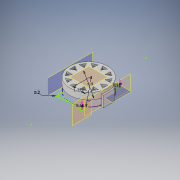
# Autodesk Inventor part: watchBodyOneTopV1.1
Saved by Autodesk Inventor 2019 (Build 230136000, 136)
## iProperties
Created: 2019-10-08
Part Number: watchBodyOneTopV1.1
Material: Generic
Document SubType Name: Modeling
Designer: Derek
Density: 1 g/cm^3
Appearance: Default
Author: Derek
Autodesk Inventor part; units mm, degrees
ref_plane "YZ Plane" through (0, 0, 0) normal (1, 0, 0) x (0, 1, 0)
ref_plane "XZ Plane" through (0, 0, 0) normal (0, 1, 0) x (-1, 0, 0)
ref_plane "XY Plane" through (0, 0, 0) normal (0, 0, 1) x (1, 0, 0)
sketch "Sketch1" plane through (0, 0, 0) normal (0, 1, 0) x (-1, 0, 0)
  circle A0 centre (0, 0) radius 22
  arc A1 (-13.7238, -17.1947) -> (13.7238, -17.1947) centre (0, 0) ccw
  dimension "d0" = 44
  dimension "d11" = 13.7238
  constraints: 4 point on circle, 2 centre point, 1 coincident, 1 concentric
  measures "d0" diameter of A0
  measures "d11" horizontal distance of point (0, 0) A0.start
ref_plane "Work Plane10" through (0, 7, 0) normal (0, 1, 0) x (1, 0, 0)
sketch "Sketch5" plane through (0, 7, 0) normal (0, 1, 0) x (1, 0, 0)
  circle A0 centre (0, 0) radius 20
  dimension "d8" = 40
  constraints: 1 centre point, 1 coincident
  measures "d8" diameter of A0
ref_plane "Work Plane9" through (0, 0, 0) normal (0, -1, 0) x (1, 0, 0)
sketch "Sketch8" plane through (0, 0, 0) normal (0, -1, 0) x (1, 0, 0)
  arc A0 (-11.5874, -18.7011) -> (11.5874, -18.7011) centre (0, 0) ccw
  line L0 (-15.0453, -16.0511) -> (-15.0453, -22.0257)
  line L1 (15.0453, -16.0511) -> (15.0453, -22.0257)
  arc A1 (-15.0453, -16.0511) -> (15.0453, -16.0511) centre (0, 0) ccw
  arc A2 (-15.0453, -22.0257) -> (-13.0453, -24.0257) centre (-13.0453, -22.0257) ccw
  arc A3 (13.0453, -24.0257) -> (15.0453, -22.0257) centre (13.0453, -22.0257) ccw
  line L2 (-15.0451, -16.0514) -> (-15.0451, -22.026)
  arc A4 (-15.0451, -22.026) -> (-13.0451, -24.026) centre (-13.0451, -22.026) ccw
  arc A5 (13.0456, -24.026) -> (15.0456, -22.026) centre (13.0456, -22.026) ccw
  line L3 (15.0456, -16.0514) -> (15.0456, -22.026)
  arc A6 (-15.0451, -16.0514) -> (15.0456, -16.0514) centre (0.0003, -0.0002) ccw
  arc A7 (13.0456, -24.026) -> (-13.0451, -24.026) centre (0.0003, -66.8475) ccw
  point P0 (0, 0)
  point P1 (0, 0)
  constraints: 16 point on circle, 8 centre point, 8 end point
ref_plane "Work Plane8" through (0, 0, 0) normal (0, -1, 0) x (1, 0, 0)
sketch "Sketch11" plane through (0, 0, 0) normal (0, -1, 0) x (1, 0, 0)
  arc A0 (11.5874, 18.7011) -> (-11.5874, 18.7011) centre (0, 0) ccw
  line L0 (-15.0453, 16.0511) -> (-15.0453, 22.0257)
  line L1 (15.0453, 16.0511) -> (15.0453, 22.0257)
  arc A1 (15.0453, 16.0511) -> (-15.0453, 16.0511) centre (0, 0) ccw
  arc A2 (-13.0453, 24.0257) -> (-15.0453, 22.0257) centre (-13.0453, 22.0257) ccw
  arc A3 (15.0453, 22.0257) -> (13.0453, 24.0257) centre (13.0453, 22.0257) ccw
  line L2 (-15.0451, 16.0514) -> (-15.0451, 22.026)
  arc A4 (-13.0451, 24.026) -> (-15.0451, 22.026) centre (-13.0451, 22.026) ccw
  arc A5 (15.0456, 22.026) -> (13.0456, 24.026) centre (13.0456, 22.026) ccw
  line L3 (15.0456, 16.0514) -> (15.0456, 22.026)
  arc A6 (15.0456, 16.0514) -> (-15.0451, 16.0514) centre (0.0003, 0.0002) ccw
  arc A7 (-13.0451, 24.026) -> (13.0456, 24.026) centre (0.0003, 66.8475) ccw
  point P0 (0, 0)
  dimension "d27" = 2
  dimension "d28" = 2
  constraints: 16 point on circle, 8 centre point, 8 end point, 4 tangent, 4 vertical, 2 equal radius
  measures "d27" radius of A2
  measures "d28" radius of A4
ref_plane "Work Plane5" through (14.0456, 0, 22.026) normal (1, 0, 0) x (0, 0, -1)
sketch "Sketch14" plane through (14.0456, 0, 22.026) normal (1, 0, 0) x (0, 0, -1)
  line L0 (0, 0) -> (0, 7) projected
  circle A0 centre (0, 3.5) radius 0.9
  point P0 (22.026, 0)
  dimension "d38" = 1.8
  constraints: 1 centre point, 1 midpoint
  measures "d38" diameter of A0
ref_plane "Work Plane6" through (14.0456, 0, 22.026) normal (1, 0, 0) x (0, 0, -1)
sketch "Sketch15" plane through (14.0456, 0, 22.026) normal (1, 0, 0) x (0, 0, -1)
  line L0 (44.1089, 7) -> (44.1089, 0) projected
  circle A0 centre (44.1089, 3.5) radius 0.9
  point P0 (22.026, 0)
  dimension "d41" = 1.8
  constraints: 1 centre point, 1 midpoint
  measures "d41" diameter of A0
ref_plane "Work Plane7" through (0, 7, 0) normal (0, 1, 0) x (1, 0, 0)
sketch "Sketch16" plane through (0, 7, 0) normal (0, 1, 0) x (1, 0, 0)
  circle A0 centre (0, 0) radius 22
  circle A1 centre (0, -0.3745) radius 18.6
  dimension "d44" = 37.2
  constraints: 2 centre point, 1 coincident
  measures "d44" diameter of A1
extrude "Extrusion13" add sketch "Sketch16" along normal blind 7.5
ref_plane "Work Plane3" through (22, 0, 0) normal (1, 0, 0) x (0, 1, 0)
sketch "Sketch17" plane through (22, 0, 0) normal (1, 0, 0) x (0, 1, 0)
  line L0 (7, -18.2255) -> (7, 18.9745) projected
  line L1 (11.1125, 6.35) -> (7, 6.35)
  line L2 (7, 6.35) -> (7, -6.5465)
  line L3 (7, -6.5465) -> (11.1125, -6.5465)
  line L4 (11.1125, -6.5465) -> (11.1125, 6.35)
  constraints: 8 end point, 2 parallel, 1 horizontal, 1 perpendicular, 1 point on line
extrude "Extrusion14" add sketch "Sketch17" along normal mid plane 3
ref_plane "Work Plane12" through (21.0034, 7, -6.5465) normal (0, -1, 0) x (1, 0, 0)
sketch "Sketch18" plane through (21.0034, 7, -6.5465) normal (0, -1, 0) x (1, 0, 0)
  arc A0 (-35.8073, -9.7276) -> (-35.8073, 22.8206) centre (-21.0034, 6.5465) ccw projected
  line L0 (0, 0) -> (2.4966, 0) projected
  line L1 (0, 0) -> (2.4966, 0)
  line L2 (2.4966, 12.8965) -> (0.0602, 12.8965) projected
  line L3 (2.4966, 0) -> (2.4966, 12.8965)
  line L4 (2.4966, 12.8965) -> (0.0602, 12.8965)
  arc A1 (0, 0) -> (0.0602, 12.8965) centre (-21.0034, 6.5465) ccw
  constraints: 6 end point, 3 point on circle, 2 collinear, 1 centre point, 1 perpendicular
extrude "Extrusion15" add sketch "Sketch18" along normal blind 8.65
ref_plane "Work Plane4" through (-22, 0, 0) normal (-1, 0, 0) x (0, -1, 0)
sketch "Sketch19" plane through (-22, 0, 0) normal (-1, 0, 0) x (0, -1, 0)
  line L0 (-11.1125, -6.5465) -> (-11.1125, 6.35) projected
  line L1 (-7, -20) -> (-7, 20) projected
  line L2 (-11.1125, -6.5465) -> (-7, -6.5465)
  line L3 (-7, -6.5465) -> (-7, 6.35)
  line L4 (-7, 6.35) -> (-11.1125, 6.35)
  line L5 (-11.1125, 6.35) -> (-11.1125, -6.5465)
  point P0 (0, 0)
  constraints: 8 end point, 2 parallel, 1 horizontal, 1 perpendicular, 1 point on line
extrude "Extrusion16" add sketch "Sketch19" along normal mid plane 3
sketch "Sketch20" plane through (-23.5, 7, -6.5465) normal (0, -1, 0) x (1, 0, 0)
  line L0 (0, 0) -> (2.4966, 0) projected
  line L1 (2.4966, 0) -> (0, 0)
  line L2 (0, 12.8965) -> (0, 0) projected
  line L3 (0, 0) -> (0, 12.8965)
  arc A0 (2.4363, 12.8965) -> (2.4966, 0) centre (23.5, 6.5465) ccw projected
  line L4 (0, 12.8965) -> (2.4363, 12.8965)
  point P0 (3, 0)
  constraints: 6 end point, 2 collinear, 1 perpendicular
extrude "Extrusion17" add sketch "Sketch20" along normal blind 8.65
sketch "Sketch21" plane through (-23.5, 0, 0) normal (-1, 0, 0) x (0, 0, 1)
  line L0 (-6.5465, 11.1125) -> (-6.5465, -1.65) projected
  line L1 (6.35, -1.65) -> (-6.5465, -1.65)
  line L2 (-6.5465, -1.65) -> (-6.5465, -0.292)
  line L3 (-6.5465, -0.292) -> (6.35, -0.292)
  line L4 (6.35, -0.292) -> (6.35, -1.65)
  point P0 (6.35, 0)
  constraints: 8 end point, 2 parallel, 1 horizontal, 1 perpendicular, 1 point on line
extrude "Extrusion18" add sketch "Sketch21" against normal blind 3.5
sketch "Sketch22" plane through (23.5, 0, 0) normal (1, 0, 0) x (0, 0, -1)
  line L0 (-6.35, -0.292) -> (6.5465, -0.292) projected
  line L1 (-6.35, -1.65) -> (6.5465, -1.65) projected
  line L2 (6.5465, -0.292) -> (-6.35, -0.292)
  line L3 (-6.35, -0.292) -> (-6.35, -1.65)
  line L4 (-6.35, -1.65) -> (6.5465, -1.65)
  line L5 (6.5465, -1.65) -> (6.5465, -0.292)
  point P0 (0, 0)
  constraints: 8 end point, 2 parallel, 1 horizontal, 1 perpendicular
extrude "Extrusion19" add sketch "Sketch22" against normal blind 3.5
ref_plane "Work Plane11" through (0, 14.5, 0) normal (0, 1, 0) x (1, 0, 0)
sketch "Sketch23" plane through (0, 14.5, 0) normal (0, 1, 0) x (1, 0, 0)
  circle A0 centre (0, 0) radius 20
  constraints: 1 centre point, 1 coincident
extrude "Extrusion20" add sketch "Sketch23" against normal blind 2
sketch "Sketch24" plane through (0, 14.5, 0) normal (0, 1, 0) x (1, 0, 0)
  line L0 (2.958, 18.9599) -> (-0.0041, 13.8437)
  line L1 (-0.0041, 13.8437) -> (-2.9538, 18.9671)
  line L2 (-2.9538, 18.9671) -> (2.958, 18.9599)
  line L3 (12.2922, 14.893) -> (7.1379, 11.9475)
  line L4 (7.1379, 11.9475) -> (7.1641, 17.884)
  line L5 (7.1641, 17.884) -> (12.2922, 14.893)
  line L6 (18.2225, 6.8835) -> (12.2004, 6.928)
  line L7 (12.2004, 6.928) -> (15.25, 12.1211)
  line L8 (15.25, 12.1211) -> (18.2225, 6.8835)
  line L9 (19.2871, 3.0371) -> (19.2959, -3.302)
  line L10 (19.2959, -3.302) -> (13.8017, -0.1401)
  line L11 (13.8017, -0.1401) -> (19.2871, 3.0371)
  line L12 (18.3039, -7.2042) -> (15.1393, -12.4356)
  line L13 (15.1393, -12.4356) -> (12.1912, -7.0793)
  line L14 (12.1912, -7.0793) -> (18.3039, -7.2042)
  line L15 (12.2922, -14.8615) -> (7.3345, -18.1476)
  line L16 (7.3345, -18.1476) -> (6.9675, -12.2111)
  line L17 (6.9675, -12.2111) -> (12.2922, -14.8615)
  line L18 (0.0704, -14.1349) -> (2.9797, -19.1738)
  line L19 (2.9797, -19.1738) -> (-2.8388, -19.1738)
  line L20 (-2.8388, -19.1738) -> (0.0704, -14.1349)
  line L21 (-7.0607, -12.1336) -> (-7.0172, -18.0963)
  line L22 (-7.0172, -18.0963) -> (-12.2028, -15.1526)
  line L23 (-12.2028, -15.1526) -> (-7.0607, -12.1336)
  line L24 (-11.9565, -7.0793) -> (-15.118, -12.5587)
  line L25 (-15.118, -12.5587) -> (-18.2826, -7.0811)
  line L26 (-18.2826, -7.0811) -> (-11.9565, -7.0793)
  line L27 (-13.7277, -0.1539) -> (-19.1828, -3.2194)
  line L28 (-19.1828, -3.2194) -> (-19.11, 3.0377)
  line L29 (-19.11, 3.0377) -> (-13.7277, -0.1539)
  line L30 (-11.9985, 6.7691) -> (-18.3039, 6.8788)
  line L31 (-18.3039, 6.8788) -> (-15.0562, 12.2846)
  line L32 (-15.0562, 12.2846) -> (-11.9985, 6.7691)
  line L33 (-7.0607, 11.7045) -> (-12.3714, 15.0155)
  line L34 (-12.3714, 15.0155) -> (-6.8486, 17.9592)
  line L35 (-6.8486, 17.9592) -> (-7.0607, 11.7045)
  point P0 (0, 0)
  point P1 (0, 17.2569)
  point P2 (8.8647, 14.9082)
  point P3 (15.2243, 8.6442)
  point P4 (17.4616, -0.135)
  point P5 (15.2115, -8.9064)
  point P6 (8.8647, -15.0734)
  point P7 (0.0704, -17.4941)
  point P8 (-8.7603, -15.1275)
  point P9 (-15.119, -8.9064)
  point P10 (-17.3402, -0.1119)
  point P11 (-15.1196, 8.6442)
  point P12 (-8.7603, 14.893)
  constraints: 72 end point, 2 point on line, 84 other
extrude "Extrusion21" cut sketch "Sketch24" against normal blind 8
body "Solid1"
